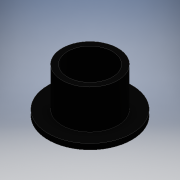
# Autodesk Inventor part: オイレス　m4　8　フランジ付き l=7
Saved by Autodesk Inventor 2016 (Build 200138000, 138)
## iProperties
Created: 2016-01-14
Part Number: オイレス　m4　8　フランジ付き l=7
Material: アセタール樹脂、黒
Document SubType Name: Modeling
Designer: Takumi
Density: 1.425 g/cm^3
Appearance: 滑らか - 黒
Mass: 0.542808 g
Surface Area: 8.34093 cm^2
Volume: 0.380918 cm^3
Author: Takumi
Autodesk Inventor part; units mm, degrees
ref_plane "YZ Plane" through (0, 0, 0) normal (1, 0, 0) x (0, 1, 0)
ref_plane "XZ Plane" through (0, 0, 0) normal (0, 1, 0) x (-1, 0, 0)
ref_plane "XY Plane" through (0, 0, 0) normal (0, 0, 1) x (1, 0, 0)
sketch "スケッチ1" plane through (0, 0, 0) normal (0, 0, 1) x (1, 0, 0)
  circle A0 centre (0, 0) radius 7.5
  circle A1 centre (0, 0) radius 5
  circle A2 centre (0, 0) radius 4
  dimension "d0" = 15
  dimension "d1" = 10
  dimension "d2" = 8
  constraints: 3 centre point, 3 coincident
  measures "d0" diameter of A0
  measures "d1" diameter of A1
  measures "d2" diameter of A2
extrude "押し出し1" add sketch "スケッチ1" along normal blind 7 contours A1
extrude "押し出し2" add sketch "スケッチ1" against normal blind 1 contours A0 | A1
